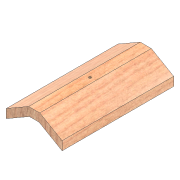
# Autodesk Inventor part: legno 2
Saved by Autodesk Inventor 2022 (Build 260153000, 153)
## iProperties
Created: 2025-08-09
Part Number: legno 2
Material: Wood (Birch)
Document SubType Name: Modeling
Designer: sacchie
Density: 0.55 g/cm^3
Appearance: Birch - Natural Polished
Author: sacchie
Autodesk Inventor part; units mm, degrees
ref_plane "YZ Plane" through (0, 0, 0) normal (1, 0, 0) x (0, 1, 0)
ref_plane "XZ Plane" through (0, 0, 0) normal (0, 1, 0) x (-1, 0, 0)
ref_plane "XY Plane" through (0, 0, 0) normal (0, 0, 1) x (1, 0, 0)
sketch "Sketch1" plane through (0, 0, 0) normal (0, 0, 1) x (1, 0, 0)
  line L0 (0, 0) -> (-20, 0)
  line L1 (-20, 0) -> (-20, 10)
  line L2 (-20, 10) -> (0, 10)
  line L3 (0, 10) -> (0, 0)
  line L4 (-10, 0) -> (-60, -28.8675)
  line L5 (-10, 0) -> (47.735, 0) construction
  line L6 (-20, 10) -> (-60, -13.094)
  line L7 (-60, -28.8675) -> (-60, -13.094)
  line L8 (-10, 0) -> (40, -28.8675)
  line L9 (-10, 0) -> (47.735, 0) construction
  line L10 (0, 10) -> (40, -13.094)
  line L11 (40, -28.8675) -> (40, -13.094)
  line L12 (-18.6603, -5) -> (-1.3397, -5)
  dimension "d0" = 20
  dimension "d1" = 10
  dimension "d7" = 150
  dimension "d8" = 50
  dimension "d9" = 30
  dimension "d10" = 50
  dimension "d11" = 5
  constraints: 26 end point, 4 horizontal, 2 equal length, 2 parallel, 2 point on line, 2 vertical, 1 midpoint, 1 perpendicular
  measures "d0" distance of L1.end L2.end
  measures "d1" distance of L0.end L1.end
  measures "d7" angle of L4 L5
  measures "d8" horizontal distance of L4.start L4.end
  measures "d9" angle of L8 L9
  measures "d10" horizontal distance of L4.start L8.end
  measures "d11" distance between parallel lines of L0 L12
extrude "Extrusion1" add sketch "Sketch1" along normal blind 200
sketch "Sketch3" plane through (-20, 10, 0) normal (0, 1, 0) x (1, 0, 0)
  line L0 (20, 0) -> (20, -200) projected
  line L1 (0, 0) -> (0, -200) construction
  line L2 (20, -200) -> (0, 0) construction
  circle A0 centre (10, -100) radius 2
  dimension "d12" = 4
  constraints: 2 end point, 1 centre point, 1 midpoint
  measures "d12" diameter of A0
extrude "Extrusion3" cut sketch "Sketch3" against normal through all
equation "\"d10\" = d8"
body "Solid1"
